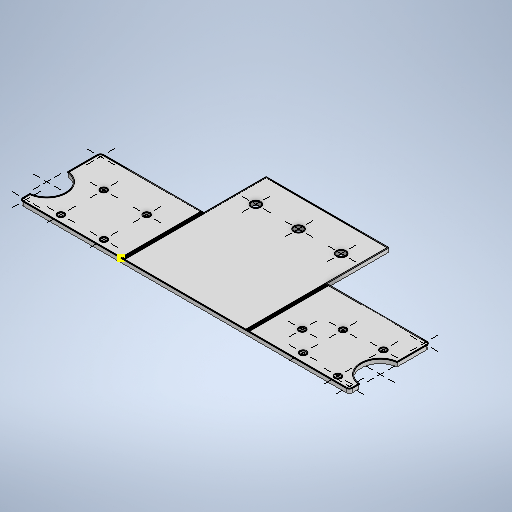
# Autodesk Inventor part: axis_22_top_frame
Saved by Autodesk Inventor 2026.1 (Build 301233000, 233)
## iProperties
Created: 2025-08-22
Part Number: axis_22_top_frame
Material: Generic
Document SubType Name: Modeling
Designer: LG
Density: 1 g/cm^3
Appearance: Default
Author: LG
Autodesk Inventor part; units mm, degrees
ref_plane "YZ Plane" through (0, 0, 0) normal (1, 0, 0) x (0, 1, 0)
ref_plane "XZ Plane" through (0, 0, 0) normal (0, 1, 0) x (-1, 0, 0)
ref_plane "XY Plane" through (0, 0, 0) normal (0, 0, 1) x (1, 0, 0)
sketch "Sketch1" plane through (0, 0, 0) normal (0, 1, 0) x (-1, 0, 0)
  line L0 (-44.2289, 0) -> (-44.2289, -28.14)
  line L1 (-0.4496, -28.14) -> (-0.4496, 0)
  circle A0 centre (23.79, -17.595) radius 1.05
  circle A1 centre (23.79, -2.545) radius 1.05
  circle A2 centre (8.69, -17.595) radius 1.05
  circle A3 centre (8.69, -2.545) radius 1.05
  circle A4 centre (-53.5486, -10.07) radius 1.05
  circle A5 centre (-60.8486, -17.07) radius 1.05
  circle A6 centre (-60.8486, -3.07) radius 1.05
  circle A7 centre (-74.0686, -18.07) radius 1.05
  circle A8 centre (-74.0686, -2.07) radius 1.05
  circle A9 centre (-37.3393, -39.96) radius 1.55
  circle A10 centre (-22.3393, -39.96) radius 1.55
  circle A11 centre (-7.3393, -39.96) radius 1.55
  arc A12 (35.49, -3.3676) -> (35.49, -16.7724) centre (36.29, -10.07) ccw
  line L2 (35.49, -1) -> (35.49, -3.3676)
  arc A13 (-80.1686, -16.7724) -> (-80.1686, -3.3676) centre (-80.9686, -10.07) ccw
  line L3 (-80.1686, -27.14) -> (-80.1686, -16.7724)
  arc A14 (-80.1686, -27.14) -> (-79.1686, -28.14) centre (-79.1686, -27.14) ccw
  line L4 (-43.7793, -28.14) -> (-79.1686, -28.14)
  line L5 (-43.7793, -50) -> (-43.7793, -28.14)
  line L6 (-0.8993, -50) -> (-43.7793, -50)
  line L7 (-0.8993, -28.14) -> (-0.8993, -50)
  line L8 (34.49, -28.14) -> (-0.8993, -28.14)
  arc A15 (34.49, -28.14) -> (35.49, -27.14) centre (34.49, -27.14) ccw
  line L9 (35.49, -16.7724) -> (35.49, -27.14)
  arc A16 (35.49, -1) -> (34.49, 0) centre (34.49, -1) ccw
  line L10 (-79.1686, 0) -> (34.49, 0)
  arc A17 (-79.1686, 0) -> (-80.1686, -1) centre (-79.1686, -1) ccw
  line L11 (-80.1686, -3.3676) -> (-80.1686, -1)
  line L12 (-44.6786, -28.14) -> (-44.6786, 0)
  line L13 (-43.7793, 0) -> (-43.7793, -28.14)
  line L14 (-0.8993, -28.14) -> (-0.8993, 0)
  line L15 (0, 0) -> (0, -28.14)
  constraints: 32 end point, 18 centre point, 14 equal radius, 12 point on circle, 12 tangent, 12 vertical, 10 parallel, 10 point on line, 4 horizontal, 3 perpendicular, 1 collinear, 63 other
extrude "Extrusion1" add sketch "Sketch1" against normal blind 1.5
body "Solid1"
